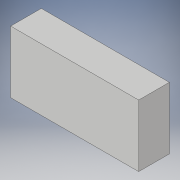
# Autodesk Inventor part: Hew Battery
Saved by Autodesk Inventor 2017 (Build 210142000, 142)
## iProperties
Created: 2016-09-27
Part Number: Hew Battery
Material: Generic
Document SubType Name: Modeling
Designer: situh
Density: 1 g/cm^3
Appearance: Default
Author: situh
Autodesk Inventor part; units mm, degrees
ref_plane "YZ Plane" through (0, 0, 0) normal (1, 0, 0) x (0, 1, 0)
ref_plane "XZ Plane" through (0, 0, 0) normal (0, 1, 0) x (-1, 0, 0)
ref_plane "XY Plane" through (0, 0, 0) normal (0, 0, 1) x (1, 0, 0)
sketch "Sketch1" plane through (0, 0, 0) normal (0, 0, 1) x (1, 0, 0)
  line L0 (-38.7411, 29.5691) -> (31.8963, 29.5691)
  line L1 (31.8963, 29.5691) -> (31.8963, -4.6193)
  line L2 (31.8963, -4.6193) -> (-38.7411, -4.6193)
  line L3 (-38.7411, -4.6193) -> (-38.7411, 29.5691)
  point P0 (0, 0)
  dimension "d0" = 70.6374
  dimension "d1" = 34.1884
  constraints: 8 end point, 2 parallel, 1 horizontal, 1 perpendicular
  measures "d0" distance of L0.start L0.end
  measures "d1" distance of L0.end L1.end
extrude "Extrusion1" add sketch "Sketch1" along normal blind 16.92
body "Solid1"
